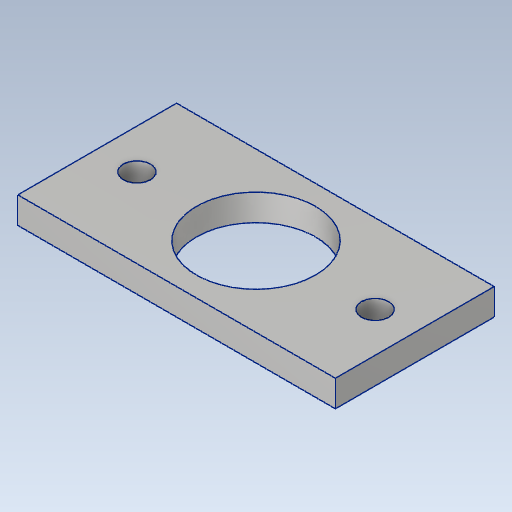
# Autodesk Inventor part: 200288
Saved by Autodesk Inventor 2020 (Build 240168000, 168)
## iProperties
Created: 2021-12-04
Part Number: 200288
Material: Aluminum 5052 H32
Document SubType Name: Sheet Metal
Designer: Byron Robotics
Mass: 37.633 g
Surface Area: 66.7207 cm^2
Volume: 13.9381 cm^3
Density: 2.7 g/cm^3
Sheet Metal Rule: .125 5052
Appearance: Aluminum - Flat
Author: Byron Robotics
Autodesk Inventor part; units mm, degrees
ref_plane "YZ Plane" through (0, 0, 0) normal (1, 0, 0) x (0, 1, 0)
ref_plane "XZ Plane" through (0, 0, 0) normal (0, 1, 0) x (-1, 0, 0)
ref_plane "XY Plane" through (0, 0, 0) normal (0, 0, 1) x (1, 0, 0)
sketch "Sketch1" plane through (0, 0, 0) normal (0, 1, 0) x (-1, 0, 0)
  line L0 (0, 0) -> (76.2, 0)
  line L1 (76.2, 0) -> (76.2, -38.1)
  line L2 (76.2, -38.1) -> (0, -38.1)
  line L3 (0, -38.1) -> (0, 0)
  dimension "d0" = 76.2
  dimension "d1" = 38.1
  measures "d0" distance of L1.end L2.end
  measures "d1" distance of L0.end L1.end
extrude "Plate1" add sketch "Sketch1" along normal blind 6.35
sketch "Sketch2" plane through (0, 6.35, 0) normal (0, 1, 0) x (1, 0, 0)
  line L0 (-76.2, 38.1) -> (0, 38.1) projected
  line L1 (-76.2, 0) -> (-76.2, 38.1) projected
  point P0 (0, 0)
  point P1 (-38.1, 19.05)
  dimension "d3" = 19.05
  dimension "d4" = 38.1
  measures "d3" distance from line of L0 point (-38.1, 19.05)
  measures "d4" distance from line of L1 point (-38.1, 19.05)
hole "Hole1" at (-38.1, 6.35, -19.05) direction (0, -1, 0) diameter 28.575 end through all
sketch "Sketch4" plane through (0, 6.35, 0) normal (0, 1, 0) x (1, 0, 0)
  line L0 (-66.675, 19.05) -> (-9.525, 19.05) construction
  circle A0 centre (-38.1, 19.05) radius 14.2875 construction
  point P0 (0, 0)
  dimension "d28" = 28.575
  dimension "d29" = 28.575
  constraints: 2 end point, 1 horizontal, 1 midpoint
  measures "d28" distance of L0.end A0.centre
  measures "d29" distance of L0.start A0.centre
hole "Hole3" at (-66.675, 6.35, -19.05) at (-9.525, 6.35, -19.05) direction (0, -1, 0) diameter 6.5278 end through all clearance for "Socket Head Cap Screw" size "1/4" standard "Ansi Unified Screw Threads"
equation "\"d4\" = 0.5 * d0"
equation "\"d10\" = Thickness"
equation "\"d28\" = CenterPointToTensionerRound"
equation "\"d29\" = d28"
equation "\"d31\" = ShapeWidth"
equation "\"d35\" = Thickness"
equation "\"d2\" = Thickness"
equation "\"BendRadius\" = 1.5 * Thickness"
equation "\"BendReliefWidth\" = Thickness"
equation "\"BendReliefDepth\" = 0.5 * Thickness"
equation "\"CornerReliefSize\" = 4 * Thickness"
equation "\"MinimumRemnant\" = 2 * Thickness"
equation "\"TransitionRadius\" = BendRadius"
equation "\"JacobiRadiusSize\" = BendRadius"
equation "\"GapSize\" = Thickness"
equation "\"DrivebaseLength\" = 762"
equation "\"DrivebaseWidth\" = 660.4"
equation "\"CenterlineDrivebaseLength\" = 736.6"
equation "\"CenterlineDrivebaseWidth\" = 635"
equation "\"ShapeHeight\" = 76.2"
equation "\"ShapeWidth\" = 25.4"
equation "\"ShapeThickness\" = 3.175"
equation "\"WheelDiameter\" = 152.4"
equation "\"WheelRadius\" = 76.2"
equation "\"WheelClearancetoFrame\" = 25.4"
equation "\"WheelDistanceFromEdge\" = 101.6"
equation "\"SlotLength\" = 88.9"
equation "\"SlotWidth\" = 15.9512"
equation "\"CenterAxleDrop\" = 3.175"
equation "\"SlidingTensionerRoundDiameter\" = 15.875"
equation "\"SlidingTensionerRoundClearance\" = 0.0762"
equation "\"CenterAxleXPosition\" = 381"
equation "\"CenterAxleYPosition\" = 25.4"
equation "\"Crossmember1Position\" = 203.2"
equation "\"Crossmember2Position\" = 203.2"
equation "\"TensionAssemblyJointTravelLengthStart\" = -15.875"
equation "\"TensionAssemblyJointTravelLengthEnd\" = 15.875"
equation "\"CenterPointToTensionerRound\" = 28.575"
equation "\"Thickness\" = 6.35"
body "Solid1"
